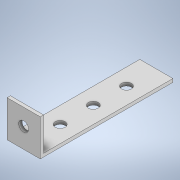
# Autodesk Inventor part: 零件1
Saved by Autodesk Inventor 2020 (Build 240168000, 168)
## iProperties
Created: 2020-10-14
Part Number: 零件1
Material: 常规
Document SubType Name: Sheet Metal
Designer: huang
Density: 1 g/cm^3
Sheet Metal Rule: 默认_mm
Appearance: 默认
Author: huang
Autodesk Inventor part; units mm, degrees
ref_plane "YZ Plane" through (0, 0, 0) normal (1, 0, 0) x (0, 1, 0)
ref_plane "XZ Plane" through (0, 0, 0) normal (0, 1, 0) x (-1, 0, 0)
ref_plane "XY Plane" through (0, 0, 0) normal (0, 0, 1) x (1, 0, 0)
sketch "草图1" plane through (0, 0, 0) normal (0, 1, 0) x (-1, 0, 0)
  line L0 (6.0123, 2.7607) -> (-3.9877, 2.7607)
  line L1 (-3.9877, 2.7607) -> (-3.9877, -37.2393)
  line L2 (-3.9877, -37.2393) -> (6.0123, -37.2393)
  line L3 (6.0123, -37.2393) -> (6.0123, 2.7607)
  point P0 (0, 0)
  dimension "d0" = 40
  dimension "d1" = 10
  constraints: 8 end point, 2 parallel, 1 horizontal, 1 perpendicular
  measures "d0" distance of L0.end L1.end
  measures "d1" distance of L0.start L0.end
extrude "拉伸1" add sketch "草图1" along normal blind 1
sketch "草图2" plane through (0, 1, 0) normal (0, 1, 0) x (1, 0, 0)
  line L0 (-6.0123, 37.2393) -> (-6.0123, -2.7607) projected
  line L1 (3.9877, -2.7607) -> (3.9877, 37.2393) projected
  line L2 (-6.0123, -2.7607) -> (3.9877, -2.7607)
  line L3 (3.9877, -2.7607) -> (3.9877, -1.7607)
  line L4 (3.9877, -1.7607) -> (-6.0123, -1.7607)
  line L5 (-6.0123, -1.7607) -> (-6.0123, -2.7607)
  point P0 (0, 0)
  point P1 (3.9877, -2.7607)
  dimension "d4" = 1
  constraints: 8 end point, 2 parallel, 1 horizontal, 1 perpendicular, 1 point on line
  measures "d4" distance of L1.start L3.end
extrude "拉伸2" add sketch "草图2" along normal blind 10
sketch "草图3" plane through (0, 11, 0) normal (0, 1, 0) x (1, 0, 0)
  line L0 (3.9877, -1.7607) -> (-6.0123, -1.7607) projected
  line L1 (-1.0123, -1.7607) -> (-1.0123, 8.2393)
  circle A0 centre (-1.0123, 8.2393) radius 1.5
  line L2 (-1.0123, 8.2393) -> (-1.0123, 18.2393)
  circle A1 centre (-1.0123, 18.2393) radius 1.5
  line L3 (-1.0123, 18.2393) -> (-1.0123, 28.2393)
  circle A2 centre (-1.0123, 28.2393) radius 1.5
  point P0 (0, 0)
  dimension "d7" = 10
  dimension "d8" = 3
  dimension "d15" = 10
  dimension "d16" = 3
  dimension "d17" = 10
  dimension "d18" = 3
  constraints: 6 end point, 3 centre point, 3 coincident, 3 vertical, 1 midpoint
  measures "d7" distance of L1.start L1.end
  measures "d8" diameter of A0
  measures "d15" distance of L2.start L2.end
  measures "d16" diameter of A1
  measures "d17" distance of L3.start L3.end
  measures "d18" diameter of A2
extrude "拉伸3" cut sketch "草图3" against normal blind 100
sketch "草图4" plane through (-6.0123, 0, 2.7607) normal (0, 0, 1) x (1, 0, 0)
  line L0 (0, 11) -> (10, 11) projected
  line L1 (5, 11) -> (5, 6)
  circle A0 centre (5, 6) radius 1.5
  point P0 (6.0123, 0)
  dimension "d11" = 5
  dimension "d12" = 3
  constraints: 2 end point, 1 centre point, 1 coincident, 1 midpoint, 1 vertical
  measures "d11" distance of L1.start L1.end
  measures "d12" diameter of A0
extrude "拉伸4" cut sketch "草图4" against normal blind 100
equation "\"折弯半径\" = 厚度"
equation "\"折弯释压宽度\" = 厚度"
equation "\"折弯释压深度\" = 0.5 * 厚度"
equation "\"拐角释压尺寸\" = 4 * 厚度"
equation "\"最小余量\" = 2 * 厚度"
equation "\"过渡半径\" = 折弯半径"
equation "\"Jacobi半径尺寸\" = 折弯半径"
equation "\"间隙大小\" = 厚度"
equation "\"厚度\" = 0.5"
